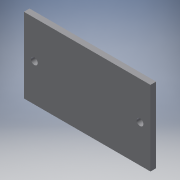
# Autodesk Inventor part: LC_mirror_holder_back
Saved by Autodesk Inventor 2019 (Build 230136000, 136)
## iProperties
Created: 2021-05-17
Part Number: LC_mirror_holder_back
Material: Generic
Document SubType Name: Modeling
Designer: UC2
Density: 1 g/cm^3
Appearance: Default
Author: UC2
Autodesk Inventor part; units mm, degrees
ref_plane "YZ Plane" through (0, 0, 0) normal (1, 0, 0) x (0, 1, 0)
ref_plane "XZ Plane" through (0, 0, 0) normal (0, 1, 0) x (-1, 0, 0)
ref_plane "XY Plane" through (0, 0, 0) normal (0, 0, 1) x (1, 0, 0)
sketch "Skizze1" plane through (0, 0, 0) normal (0, 0, 1) x (1, 0, 0)
  line L0 (-38.99, 0) -> (38.99, 0) construction
  line L1 (0, -23.1) -> (0, 23.1) construction
  line L2 (-27.85, -16.5) -> (27.85, -16.5)
  line L3 (27.85, -16.5) -> (27.85, 16.5)
  line L4 (27.85, 16.5) -> (-27.85, 16.5)
  line L5 (-27.85, 16.5) -> (-27.85, -16.5)
  line L6 (-27.85, -16.5) -> (27.85, 16.5) construction
  line L7 (27.85, -16.5) -> (-27.85, 16.5) construction
  line L8 (-26.75, -16.5) -> (26.75, -16.5) construction
  line L9 (26.75, -16.5) -> (26.75, 16.5) construction
  line L10 (26.75, 16.5) -> (-26.75, 16.5) construction
  line L11 (-26.75, 16.5) -> (-26.75, -16.5) construction
  line L12 (-26.75, -16.5) -> (26.75, 16.5) construction
  line L13 (26.75, -16.5) -> (-26.75, 16.5) construction
  circle A0 centre (-23.25, -8.25) radius 1.5
  circle A1 centre (23.25, -8.25) radius 1.5
  circle A2 centre (-23.25, 8.25) radius 1.5
  circle A3 centre (23.25, 8.25) radius 1.5
  point P0 (0, 0)
  dimension "d0" = 55.7
  dimension "d1" = 33
  dimension "d4" = 53.5
  dimension "d5" = 3
  dimension "d9" = 8.25
  dimension "d10" = 23.25
  constraints: 24 end point, 4 centre point, 4 midpoint, 4 parallel, 3 symmetric about line, 2 horizontal, 2 perpendicular, 1 point on line, 3 other
  measures "d0" distance of L3.end L4.end
  measures "d1" distance of L2.end L3.end
  measures "d4" distance of L10.end L9.end
  measures "d5" diameter of A0
  measures "d9" distance from line of L8 A0.centre
  measures "d10" distance from line of L1 A0.centre
extrude "Extrusion1" add sketch "Skizze1" along normal blind 2.5
